Autodesk Fusion 360 part; units mm, degrees
(part 5 of 40)
  line L1833 (198.3385, 89.2864) -> (198.2749, 89.1443) construction
  line L1834 (198.2749, 89.1443) -> (198.2094, 89.0029) construction
  line L1835 (198.2094, 89.0029) -> (198.1418, 88.8621) construction
  line L1836 (198.1418, 88.8621) -> (198.072, 88.7221) construction
  line L1837 (198.072, 88.7221) -> (198.0004, 88.5827) construction
  line L1838 (198.0004, 88.5827) -> (197.927, 88.4439) construction
  line L1839 (197.927, 88.4439) -> (197.8523, 88.3056) construction
  line L1840 (197.8523, 88.3056) -> (197.7763, 88.1678) construction
  line L1841 (197.7763, 88.1678) -> (197.6993, 88.0303) construction
  line L1842 (197.6993, 88.0303) -> (197.6211, 87.8933) construction
  line L1843 (197.6211, 87.8933) -> (197.5416, 87.7568) construction
  line L1844 (197.5416, 87.7568) -> (197.4609, 87.6208) construction
  line L1845 (197.4609, 87.6208) -> (197.379, 87.4852) construction
  line L1846 (197.379, 87.4852) -> (197.2957, 87.3502) construction
  line L1847 (197.2957, 87.3502) -> (197.2112, 87.2157) construction
  line L1848 (197.2112, 87.2157) -> (197.1256, 87.0816) construction
  line L1849 (197.1256, 87.0816) -> (197.0388, 86.948) construction
  line L1850 (197.0388, 86.948) -> (196.951, 86.8148) construction
  line L1851 (196.951, 86.8148) -> (196.8622, 86.682) construction
  line L1852 (196.8622, 86.682) -> (196.7723, 86.5497) construction
  line L1853 (196.7723, 86.5497) -> (196.6814, 86.4179) construction
  line L1854 (196.6814, 86.4179) -> (196.5895, 86.2865) construction
  line L1855 (196.5895, 86.2865) -> (196.4966, 86.1555) construction
  line L1856 (196.4966, 86.1555) -> (196.4027, 86.025) construction
  line L1857 (196.4027, 86.025) -> (196.3078, 85.895) construction
  line L1858 (196.3078, 85.895) -> (196.212, 85.7654) construction
  line L1859 (196.212, 85.7654) -> (196.1152, 85.6362) construction
  line L1860 (196.1152, 85.6362) -> (196.0174, 85.5074) construction
  line L1861 (196.0174, 85.5074) -> (195.9188, 85.3791) construction
  line L1862 (195.9188, 85.3791) -> (195.8193, 85.2512) construction
  line L1863 (195.8193, 85.2512) -> (195.7189, 85.1238) construction
  line L1864 (195.7189, 85.1238) -> (195.6176, 84.9968) construction
  line L1865 (195.6176, 84.9968) -> (195.5154, 84.8702) construction
  line L1866 (195.5154, 84.8702) -> (195.4124, 84.744) construction
  line L1867 (195.4124, 84.744) -> (195.3085, 84.6183) construction
  line L1868 (195.3085, 84.6183) -> (195.2037, 84.493) construction
  line L1869 (195.2037, 84.493) -> (195.0982, 84.3682) construction
  line L1870 (195.0982, 84.3682) -> (194.9918, 84.2438) construction
  line L1871 (194.9918, 84.2438) -> (194.8846, 84.1198) construction
  line L1872 (194.8846, 84.1198) -> (194.7765, 83.9962) construction
  line L1873 (194.7765, 83.9962) -> (194.6677, 83.8731) construction
  line L1874 (194.6677, 83.8731) -> (194.5581, 83.7503) construction
  line L1875 (194.5581, 83.7503) -> (194.4478, 83.6281) construction
  line L1876 (194.4478, 83.6281) -> (194.3366, 83.5062) construction
  line L1877 (194.3366, 83.5062) -> (194.2247, 83.3848) construction
  line L1878 (194.2247, 83.3848) -> (194.112, 83.2638) construction
  line L1879 (194.112, 83.2638) -> (193.9985, 83.1432) construction
  line L1880 (193.9985, 83.1432) -> (193.8843, 83.0231) construction
  line L1881 (193.8843, 83.0231) -> (193.7694, 82.9034) construction
  line L1882 (193.7694, 82.9034) -> (193.6538, 82.7841) construction
  line L1883 (193.6538, 82.7841) -> (193.5374, 82.6653) construction
  line L1884 (193.5374, 82.6653) -> (193.4202, 82.5469) construction
  line L1885 (193.4202, 82.5469) -> (193.3024, 82.4289) construction
  line L1886 (193.3024, 82.4289) -> (193.1839, 82.3113) construction
  line L1887 (193.1839, 82.3113) -> (193.0646, 82.1942) construction
  line L1888 (193.0646, 82.1942) -> (192.9447, 82.0775) construction
  line L1889 (192.9447, 82.0775) -> (192.8241, 81.9612) construction
  line L1890 (192.8241, 81.9612) -> (192.7027, 81.8454) construction
  line L1891 (192.7027, 81.8454) -> (192.5808, 81.73) construction
  line L1892 (192.5808, 81.73) -> (192.4581, 81.615) construction
  line L1893 (192.4581, 81.615) -> (192.3594, 81.5233) construction
  line L1894 (192.3594, 81.5233) -> (192.2851, 81.4548) construction
  line L1895 (192.2851, 81.4548) -> (192.2354, 81.4092) construction
  line L1896 (192.2354, 81.4092) -> (192.2105, 81.3864) construction
  spline S25 degree 5 poles (198.7698, 90.4458) (198.763, 90.4157) (198.7487, 90.3556) (198.7249, 90.2662) (198.6885, 90.1483) (198.6369, 90.0027) (198.5809, 89.8584) (198.5221, 89.7148) (198.4619, 89.5717) (198.4007, 89.4289) (198.3385, 89.2864) (198.2749, 89.1443) (198.2094, 89.0029) (198.1418, 88.8621) (198.072, 88.7221) (198.0004, 88.5827) (197.927, 88.4439) (197.8523, 88.3056) (197.7763, 88.1678) (197.6993, 88.0303) (197.6211, 87.8933) (197.5416, 87.7568) (197.4609, 87.6208) (197.379, 87.4852) (197.2957, 87.3502) (197.2112, 87.2157) (197.1256, 87.0816) (197.0388, 86.948) (196.951, 86.8148) (196.8622, 86.682) (196.7723, 86.5497) (196.6814, 86.4179) (196.5895, 86.2865) (196.4966, 86.1555) (196.4027, 86.025) (196.3078, 85.895) (196.212, 85.7654) (196.1152, 85.6362) (196.0174, 85.5074) (195.9188, 85.3791) (195.8193, 85.2512) (195.7189, 85.1238) (195.6176, 84.9968) (195.5154, 84.8702) (195.4124, 84.744) (195.3085, 84.6183) (195.2037, 84.493) (195.0982, 84.3682) (194.9918, 84.2438) (194.8846, 84.1198) (194.7765, 83.9962) (194.6677, 83.8731) (194.5581, 83.7503) (194.4478, 83.6281) (194.3366, 83.5062) (194.2247, 83.3848) (194.112, 83.2638) (193.9985, 83.1432) (193.8843, 83.0231) (193.7694, 82.9034) (193.6538, 82.7841) (193.5374, 82.6653) (193.4202, 82.5469) (193.3024, 82.4289) (193.1839, 82.3113) (193.0646, 82.1942) (192.9447, 82.0775) (192.8241, 81.9612) (192.7027, 81.8454) (192.5808, 81.73) (192.4581, 81.615) (192.3594, 81.5233) (192.2851, 81.4548) (192.2354, 81.4092) (192.2105, 81.3864) knots 0 0 0 0 0 0 0.01428571 0.02857143 0.04285714 0.05714286 0.07142857 0.08571429 0.1 0.11428571 0.12857143 0.14285714 0.15714286 0.17142857 0.18571429 0.2 0.21428571 0.22857143 0.24285714 0.25714286 0.27142857 0.28571429 0.3 0.31428571 0.32857143 0.34285714 0.35714286 0.37142857 0.38571429 0.4 0.41428571 0.42857143 0.44285714 0.45714286 0.47142857 0.48571429 0.5 0.51428571 0.52857143 0.54285714 0.55714286 0.57142857 0.58571429 0.6 0.61428571 0.62857143 0.64285714 0.65714286 0.67142857 0.68571429 0.7 0.71428571 0.72857143 0.74285714 0.75714286 0.77142857 0.78571429 0.8 0.81428571 0.82857143 0.84285714 0.85714286 0.87142857 0.88571429 0.9 0.91428571 0.92857143 0.94285714 0.95714286 0.97142857 0.98571429 1 1 1 1 1 1
  line L1897 (198.7698, 90.4458) -> (198.763, 90.4157) construction
  line L1898 (198.763, 90.4157) -> (198.7487, 90.3556) construction
  line L1899 (198.7487, 90.3556) -> (198.7249, 90.2662) construction
  line L1900 (198.7249, 90.2662) -> (198.6885, 90.1483) construction
  line L1901 (198.6885, 90.1483) -> (198.6369, 90.0027) construction
  line L1902 (198.6369, 90.0027) -> (198.5809, 89.8584) construction
  line L1903 (198.5809, 89.8584) -> (198.5221, 89.7148) construction
  line L1904 (198.5221, 89.7148) -> (198.4619, 89.5717) construction
  line L1905 (198.4619, 89.5717) -> (198.4007, 89.4289) construction
  line L1906 (198.4007, 89.4289) -> (198.3385, 89.2864) construction
  line L1907 (198.3385, 89.2864) -> (198.2749, 89.1443) construction
  line L1908 (198.2749, 89.1443) -> (198.2094, 89.0029) construction
  line L1909 (198.2094, 89.0029) -> (198.1418, 88.8621) construction
  line L1910 (198.1418, 88.8621) -> (198.072, 88.7221) construction
  line L1911 (198.072, 88.7221) -> (198.0004, 88.5827) construction
  line L1912 (198.0004, 88.5827) -> (197.927, 88.4439) construction
  line L1913 (197.927, 88.4439) -> (197.8523, 88.3056) construction
  line L1914 (197.8523, 88.3056) -> (197.7763, 88.1678) construction
  line L1915 (197.7763, 88.1678) -> (197.6993, 88.0303) construction
  line L1916 (197.6993, 88.0303) -> (197.6211, 87.8933) construction
  line L1917 (197.6211, 87.8933) -> (197.5416, 87.7568) construction
  line L1918 (197.5416, 87.7568) -> (197.4609, 87.6208) construction
  line L1919 (197.4609, 87.6208) -> (197.379, 87.4852) construction
  line L1920 (197.379, 87.4852) -> (197.2957, 87.3502) construction
  line L1921 (197.2957, 87.3502) -> (197.2112, 87.2157) construction
  line L1922 (197.2112, 87.2157) -> (197.1256, 87.0816) construction
  line L1923 (197.1256, 87.0816) -> (197.0388, 86.948) construction
  line L1924 (197.0388, 86.948) -> (196.951, 86.8148) construction
  line L1925 (196.951, 86.8148) -> (196.8622, 86.682) construction
  line L1926 (196.8622, 86.682) -> (196.7723, 86.5497) construction
  line L1927 (196.7723, 86.5497) -> (196.6814, 86.4179) construction
  line L1928 (196.6814, 86.4179) -> (196.5895, 86.2865) construction
  line L1929 (196.5895, 86.2865) -> (196.4966, 86.1555) construction
  line L1930 (196.4966, 86.1555) -> (196.4027, 86.025) construction
  line L1931 (196.4027, 86.025) -> (196.3078, 85.895) construction
  line L1932 (196.3078, 85.895) -> (196.212, 85.7654) construction
  line L1933 (196.212, 85.7654) -> (196.1152, 85.6362) construction
  line L1934 (196.1152, 85.6362) -> (196.0174, 85.5074) construction
  line L1935 (196.0174, 85.5074) -> (195.9188, 85.3791) construction
  line L1936 (195.9188, 85.3791) -> (195.8193, 85.2512) construction
  line L1937 (195.8193, 85.2512) -> (195.7189, 85.1238) construction
  line L1938 (195.7189, 85.1238) -> (195.6176, 84.9968) construction
  line L1939 (195.6176, 84.9968) -> (195.5154, 84.8702) construction
  line L1940 (195.5154, 84.8702) -> (195.4124, 84.744) construction
  line L1941 (195.4124, 84.744) -> (195.3085, 84.6183) construction
  line L1942 (195.3085, 84.6183) -> (195.2037, 84.493) construction
  line L1943 (195.2037, 84.493) -> (195.0982, 84.3682) construction
  line L1944 (195.0982, 84.3682) -> (194.9918, 84.2438) construction
  line L1945 (194.9918, 84.2438) -> (194.8846, 84.1198) construction
  line L1946 (194.8846, 84.1198) -> (194.7765, 83.9962) construction
  line L1947 (194.7765, 83.9962) -> (194.6677, 83.8731) construction
  line L1948 (194.6677, 83.8731) -> (194.5581, 83.7503) construction
  line L1949 (194.5581, 83.7503) -> (194.4478, 83.6281) construction
  line L1950 (194.4478, 83.6281) -> (194.3366, 83.5062) construction
  line L1951 (194.3366, 83.5062) -> (194.2247, 83.3848) construction
  line L1952 (194.2247, 83.3848) -> (194.112, 83.2638) construction
  line L1953 (194.112, 83.2638) -> (193.9985, 83.1432) construction
  line L1954 (193.9985, 83.1432) -> (193.8843, 83.0231) construction
  line L1955 (193.8843, 83.0231) -> (193.7694, 82.9034) construction
  line L1956 (193.7694, 82.9034) -> (193.6538, 82.7841) construction
  line L1957 (193.6538, 82.7841) -> (193.5374, 82.6653) construction
  line L1958 (193.5374, 82.6653) -> (193.4202, 82.5469) construction
  line L1959 (193.4202, 82.5469) -> (193.3024, 82.4289) construction
  line L1960 (193.3024, 82.4289) -> (193.1839, 82.3113) construction
  line L1961 (193.1839, 82.3113) -> (193.0646, 82.1942) construction
  line L1962 (193.0646, 82.1942) -> (192.9447, 82.0775) construction
  line L1963 (192.9447, 82.0775) -> (192.8241, 81.9612) construction
  line L1964 (192.8241, 81.9612) -> (192.7027, 81.8454) construction
  line L1965 (192.7027, 81.8454) -> (192.5808, 81.73) construction
  line L1966 (192.5808, 81.73) -> (192.4581, 81.615) construction
  line L1967 (192.4581, 81.615) -> (192.3594, 81.5233) construction
  line L1968 (192.3594, 81.5233) -> (192.2851, 81.4548) construction
  line L1969 (192.2851, 81.4548) -> (192.2354, 81.4092) construction
  line L1970 (192.2354, 81.4092) -> (192.2105, 81.3864) construction
  arc A68 (170.3188, 110.6216) -> (167.5414, 110.7517) centre (168.8628, 109.2504) ccw
  arc A69 (184.5338, 99.6279) -> (187.6019, 98.0646) centre (212.132, 150) ccw
  line L1971 (188.5839, 95.4634) -> (187.9372, 93.9655)
  arc A70 (199.127, 207.9623) -> (201.4504, 206.435) centre (201.0785, 208.4001) ccw
  line L1972 (188.5839, 95.4634) -> (187.9372, 93.9655)
  arc A71 (184.5338, 99.6279) -> (187.6019, 98.0646) centre (212.132, 150) ccw
  spline S26 degree 5 poles (198.7698, 209.5542) (198.763, 209.5843) (198.7487, 209.6444) (198.7249, 209.7338) (198.6885, 209.8517) (198.6369, 209.9973) (198.5809, 210.1416) (198.5221, 210.2852) (198.4619, 210.4283) (198.4007, 210.5711) (198.3385, 210.7136) (198.2749, 210.8557) (198.2094, 210.9971) (198.1418, 211.1379) (198.072, 211.2779) (198.0004, 211.4173) (197.927, 211.5561) (197.8523, 211.6944) (197.7763, 211.8322) (197.6993, 211.9697) (197.6211, 212.1067) (197.5416, 212.2432) (197.4609, 212.3792) (197.379, 212.5148) (197.2957, 212.6498) (197.2112, 212.7843) (197.1256, 212.9184) (197.0388, 213.052) (196.951, 213.1852) (196.8622, 213.318) (196.7723, 213.4503) (196.6814, 213.5821) (196.5895, 213.7135) (196.4966, 213.8445) (196.4027, 213.975) (196.3078, 214.105) (196.212, 214.2346) (196.1152, 214.3638) (196.0174, 214.4926) (195.9188, 214.6209) (195.8193, 214.7488) (195.7189, 214.8762) (195.6176, 215.0032) (195.5154, 215.1298) (195.4124, 215.256) (195.3085, 215.3817) (195.2037, 215.507) (195.0982, 215.6318) (194.9918, 215.7562) (194.8846, 215.8802) (194.7765, 216.0038) (194.6677, 216.1269) (194.5581, 216.2497) (194.4478, 216.3719) (194.3366, 216.4938) (194.2247, 216.6152) (194.112, 216.7362) (193.9985, 216.8568) (193.8843, 216.9769) (193.7694, 217.0966) (193.6538, 217.2159) (193.5374, 217.3347) (193.4202, 217.4531) (193.3024, 217.5711) (193.1839, 217.6887) (193.0646, 217.8058) (192.9447, 217.9225) (192.8241, 218.0388) (192.7027, 218.1546) (192.5808, 218.27) (192.4581, 218.385) (192.3594, 218.4767) (192.2851, 218.5452) (192.2354, 218.5908) (192.2105, 218.6136) knots 0 0 0 0 0 0 0.01428571 0.02857143 0.04285714 0.05714286 0.07142857 0.08571429 0.1 0.11428571 0.12857143 0.14285714 0.15714286 0.17142857 0.18571429 0.2 0.21428571 0.22857143 0.24285714 0.25714286 0.27142857 0.28571429 0.3 0.31428571 0.32857143 0.34285714 0.35714286 0.37142857 0.38571429 0.4 0.41428571 0.42857143 0.44285714 0.45714286 0.47142857 0.48571429 0.5 0.51428571 0.52857143 0.54285714 0.55714286 0.57142857 0.58571429 0.6 0.61428571 0.62857143 0.64285714 0.65714286 0.67142857 0.68571429 0.7 0.71428571 0.72857143 0.74285714 0.75714286 0.77142857 0.78571429 0.8 0.81428571 0.82857143 0.84285714 0.85714286 0.87142857 0.88571429 0.9 0.91428571 0.92857143 0.94285714 0.95714286 0.97142857 0.98571429 1 1 1 1 1 1
  line L1973 (198.7698, 209.5542) -> (198.763, 209.5843) construction
  line L1974 (198.763, 209.5843) -> (198.7487, 209.6444) construction
  line L1975 (198.7487, 209.6444) -> (198.7249, 209.7338) construction
  line L1976 (198.7249, 209.7338) -> (198.6885, 209.8517) construction
  line L1977 (198.6885, 209.8517) -> (198.6369, 209.9973) construction
  line L1978 (198.6369, 209.9973) -> (198.5809, 210.1416) construction
  line L1979 (198.5809, 210.1416) -> (198.5221, 210.2852) construction
  line L1980 (198.5221, 210.2852) -> (198.4619, 210.4283) construction
  line L1981 (198.4619, 210.4283) -> (198.4007, 210.5711) construction
  line L1982 (198.4007, 210.5711) -> (198.3385, 210.7136) construction
  line L1983 (198.3385, 210.7136) -> (198.2749, 210.8557) construction
  line L1984 (198.2749, 210.8557) -> (198.2094, 210.9971) construction
  line L1985 (198.2094, 210.9971) -> (198.1418, 211.1379) construction
  line L1986 (198.1418, 211.1379) -> (198.072, 211.2779) construction
  line L1987 (198.072, 211.2779) -> (198.0004, 211.4173) construction
  line L1988 (198.0004, 211.4173) -> (197.927, 211.5561) construction
  line L1989 (197.927, 211.5561) -> (197.8523, 211.6944) construction
  line L1990 (197.8523, 211.6944) -> (197.7763, 211.8322) construction
  line L1991 (197.7763, 211.8322) -> (197.6993, 211.9697) construction
  line L1992 (197.6993, 211.9697) -> (197.6211, 212.1067) construction
  line L1993 (197.6211, 212.1067) -> (197.5416, 212.2432) construction
  line L1994 (197.5416, 212.2432) -> (197.4609, 212.3792) construction
  line L1995 (197.4609, 212.3792) -> (197.379, 212.5148) construction
  line L1996 (197.379, 212.5148) -> (197.2957, 212.6498) construction
  line L1997 (197.2957, 212.6498) -> (197.2112, 212.7843) construction
  line L1998 (197.2112, 212.7843) -> (197.1256, 212.9184) construction
  line L1999 (197.1256, 212.9184) -> (197.0388, 213.052) construction
  line L2000 (197.0388, 213.052) -> (196.951, 213.1852) construction
  line L2001 (196.951, 213.1852) -> (196.8622, 213.318) construction
  line L2002 (196.8622, 213.318) -> (196.7723, 213.4503) construction
  line L2003 (196.7723, 213.4503) -> (196.6814, 213.5821) construction
  line L2004 (196.6814, 213.5821) -> (196.5895, 213.7135) construction
  line L2005 (196.5895, 213.7135) -> (196.4966, 213.8445) construction
  line L2006 (196.4966, 213.8445) -> (196.4027, 213.975) construction
  line L2007 (196.4027, 213.975) -> (196.3078, 214.105) construction
  line L2008 (196.3078, 214.105) -> (196.212, 214.2346) construction
  line L2009 (196.212, 214.2346) -> (196.1152, 214.3638) construction
  line L2010 (196.1152, 214.3638) -> (196.0174, 214.4926) construction
  line L2011 (196.0174, 214.4926) -> (195.9188, 214.6209) construction
  line L2012 (195.9188, 214.6209) -> (195.8193, 214.7488) construction
  line L2013 (195.8193, 214.7488) -> (195.7189, 214.8762) construction
  line L2014 (195.7189, 214.8762) -> (195.6176, 215.0032) construction
  line L2015 (195.6176, 215.0032) -> (195.5154, 215.1298) construction
  line L2016 (195.5154, 215.1298) -> (195.4124, 215.256) construction
  line L2017 (195.4124, 215.256) -> (195.3085, 215.3817) construction
  line L2018 (195.3085, 215.3817) -> (195.2037, 215.507) construction
  line L2019 (195.2037, 215.507) -> (195.0982, 215.6318) construction
  line L2020 (195.0982, 215.6318) -> (194.9918, 215.7562) construction
  line L2021 (194.9918, 215.7562) -> (194.8846, 215.8802) construction
  line L2022 (194.8846, 215.8802) -> (194.7765, 216.0038) construction
  line L2023 (194.7765, 216.0038) -> (194.6677, 216.1269) construction
  line L2024 (194.6677, 216.1269) -> (194.5581, 216.2497) construction
  line L2025 (194.5581, 216.2497) -> (194.4478, 216.3719) construction
  line L2026 (194.4478, 216.3719) -> (194.3366, 216.4938) construction
  line L2027 (194.3366, 216.4938) -> (194.2247, 216.6152) construction
  line L2028 (194.2247, 216.6152) -> (194.112, 216.7362) construction
  line L2029 (194.112, 216.7362) -> (193.9985, 216.8568) construction
  line L2030 (193.9985, 216.8568) -> (193.8843, 216.9769) construction
  line L2031 (193.8843, 216.9769) -> (193.7694, 217.0966) construction
  line L2032 (193.7694, 217.0966) -> (193.6538, 217.2159) construction
  line L2033 (193.6538, 217.2159) -> (193.5374, 217.3347) construction
  line L2034 (193.5374, 217.3347) -> (193.4202, 217.4531) construction
  line L2035 (193.4202, 217.4531) -> (193.3024, 217.5711) construction
  line L2036 (193.3024, 217.5711) -> (193.1839, 217.6887) construction
  line L2037 (193.1839, 217.6887) -> (193.0646, 217.8058) construction
  line L2038 (193.0646, 217.8058) -> (192.9447, 217.9225) construction
  line L2039 (192.9447, 217.9225) -> (192.8241, 218.0388) construction
  line L2040 (192.8241, 218.0388) -> (192.7027, 218.1546) construction
  line L2041 (192.7027, 218.1546) -> (192.5808, 218.27) construction
  line L2042 (192.5808, 218.27) -> (192.4581, 218.385) construction
  line L2043 (192.4581, 218.385) -> (192.3594, 218.4767) construction
  line L2044 (192.3594, 218.4767) -> (192.2851, 218.5452) construction
  line L2045 (192.2851, 218.5452) -> (192.2354, 218.5908) construction
  line L2046 (192.2354, 218.5908) -> (192.2105, 218.6136) construction
  arc A72 (188.5839, 95.4634) -> (187.6019, 98.0646) centre (186.7478, 96.2562) ccw
  spline S27 degree 5 poles (198.7698, 209.5542) (198.763, 209.5843) (198.7487, 209.6444) (198.7249, 209.7338) (198.6885, 209.8517) (198.6369, 209.9973) (198.5809, 210.1416) (198.5221, 210.2852) (198.4619, 210.4283) (198.4007, 210.5711) (198.3385, 210.7136) (198.2749, 210.8557) (198.2094, 210.9971) (198.1418, 211.1379) (198.072, 211.2779) (198.0004, 211.4173) (197.927, 211.5561) (197.8523, 211.6944) (197.7763, 211.8322) (197.6993, 211.9697) (197.6211, 212.1067) (197.5416, 212.2432) (197.4609, 212.3792) (197.379, 212.5148) (197.2957, 212.6498) (197.2112, 212.7843) (197.1256, 212.9184) (197.0388, 213.052) (196.951, 213.1852) (196.8622, 213.318) (196.7723, 213.4503) (196.6814, 213.5821) (196.5895, 213.7135) (196.4966, 213.8445) (196.4027, 213.975) (196.3078, 214.105) (196.212, 214.2346) (196.1152, 214.3638) (196.0174, 214.4926) (195.9188, 214.6209) (195.8193, 214.7488) (195.7189, 214.8762) (195.6176, 215.0032) (195.5154, 215.1298) (195.4124, 215.256) (195.3085, 215.3817) (195.2037, 215.507) (195.0982, 215.6318) (194.9918, 215.7562) (194.8846, 215.8802) (194.7765, 216.0038) (194.6677, 216.1269) (194.5581, 216.2497) (194.4478, 216.3719) (194.3366, 216.4938) (194.2247, 216.6152) (194.112, 216.7362) (193.9985, 216.8568) (193.8843, 216.9769) (193.7694, 217.0966) (193.6538, 217.2159) (193.5374, 217.3347) (193.4202, 217.4531) (193.3024, 217.5711) (193.1839, 217.6887) (193.0646, 217.8058) (192.9447, 217.9225) (192.8241, 218.0388) (192.7027, 218.1546) (192.5808, 218.27) (192.4581, 218.385) (192.3594, 218.4767) (192.2851, 218.5452) (192.2354, 218.5908) (192.2105, 218.6136) knots 0 0 0 0 0 0 0.01428571 0.02857143 0.04285714 0.05714286 0.07142857 0.08571429 0.1 0.11428571 0.12857143 0.14285714 0.15714286 0.17142857 0.18571429 0.2 0.21428571 0.22857143 0.24285714 0.25714286 0.27142857 0.28571429 0.3 0.31428571 0.32857143 0.34285714 0.35714286 0.37142857 0.38571429 0.4 0.41428571 0.42857143 0.44285714 0.45714286 0.47142857 0.48571429 0.5 0.51428571 0.52857143 0.54285714 0.55714286 0.57142857 0.58571429 0.6 0.61428571 0.62857143 0.64285714 0.65714286 0.67142857 0.68571429 0.7 0.71428571 0.72857143 0.74285714 0.75714286 0.77142857 0.78571429 0.8 0.81428571 0.82857143 0.84285714 0.85714286 0.87142857 0.88571429 0.9 0.91428571 0.92857143 0.94285714 0.95714286 0.97142857 0.98571429 1 1 1 1 1 1
  line L2047 (198.7698, 209.5542) -> (198.763, 209.5843) construction
  line L2048 (198.763, 209.5843) -> (198.7487, 209.6444) construction
  line L2049 (198.7487, 209.6444) -> (198.7249, 209.7338) construction
  line L2050 (198.7249, 209.7338) -> (198.6885, 209.8517) construction
  line L2051 (198.6885, 209.8517) -> (198.6369, 209.9973) construction
  line L2052 (198.6369, 209.9973) -> (198.5809, 210.1416) construction
  line L2053 (198.5809, 210.1416) -> (198.5221, 210.2852) construction
  line L2054 (198.5221, 210.2852) -> (198.4619, 210.4283) construction
  line L2055 (198.4619, 210.4283) -> (198.4007, 210.5711) construction
  line L2056 (198.4007, 210.5711) -> (198.3385, 210.7136) construction
  line L2057 (198.3385, 210.7136) -> (198.2749, 210.8557) construction
  line L2058 (198.2749, 210.8557) -> (198.2094, 210.9971) construction
  line L2059 (198.2094, 210.9971) -> (198.1418, 211.1379) construction
  line L2060 (198.1418, 211.1379) -> (198.072, 211.2779) construction
  line L2061 (198.072, 211.2779) -> (198.0004, 211.4173) construction
  line L2062 (198.0004, 211.4173) -> (197.927, 211.5561) construction
  line L2063 (197.927, 211.5561) -> (197.8523, 211.6944) construction
  line L2064 (197.8523, 211.6944) -> (197.7763, 211.8322) construction
  line L2065 (197.7763, 211.8322) -> (197.6993, 211.9697) construction
  line L2066 (197.6993, 211.9697) -> (197.6211, 212.1067) construction
  line L2067 (197.6211, 212.1067) -> (197.5416, 212.2432) construction
  line L2068 (197.5416, 212.2432) -> (197.4609, 212.3792) construction
  line L2069 (197.4609, 212.3792) -> (197.379, 212.5148) construction
  line L2070 (197.379, 212.5148) -> (197.2957, 212.6498) construction
  line L2071 (197.2957, 212.6498) -> (197.2112, 212.7843) construction
  line L2072 (197.2112, 212.7843) -> (197.1256, 212.9184) construction
  line L2073 (197.1256, 212.9184) -> (197.0388, 213.052) construction
  line L2074 (197.0388, 213.052) -> (196.951, 213.1852) construction
  line L2075 (196.951, 213.1852) -> (196.8622, 213.318) construction
  line L2076 (196.8622, 213.318) -> (196.7723, 213.4503) construction
  line L2077 (196.7723, 213.4503) -> (196.6814, 213.5821) construction
  line L2078 (196.6814, 213.5821) -> (196.5895, 213.7135) construction
  line L2079 (196.5895, 213.7135) -> (196.4966, 213.8445) construction
  line L2080 (196.4966, 213.8445) -> (196.4027, 213.975) construction
  line L2081 (196.4027, 213.975) -> (196.3078, 214.105) construction
  line L2082 (196.3078, 214.105) -> (196.212, 214.2346) construction
  line L2083 (196.212, 214.2346) -> (196.1152, 214.3638) construction
  line L2084 (196.1152, 214.3638) -> (196.0174, 214.4926) construction
  line L2085 (196.0174, 214.4926) -> (195.9188, 214.6209) construction
  line L2086 (195.9188, 214.6209) -> (195.8193, 214.7488) construction
  line L2087 (195.8193, 214.7488) -> (195.7189, 214.8762) construction
  line L2088 (195.7189, 214.8762) -> (195.6176, 215.0032) construction
  line L2089 (195.6176, 215.0032) -> (195.5154, 215.1298) construction
  line L2090 (195.5154, 215.1298) -> (195.4124, 215.256) construction
  line L2091 (195.4124, 215.256) -> (195.3085, 215.3817) construction
  line L2092 (195.3085, 215.3817) -> (195.2037, 215.507) construction
  line L2093 (195.2037, 215.507) -> (195.0982, 215.6318) construction
  line L2094 (195.0982, 215.6318) -> (194.9918, 215.7562) construction
  line L2095 (194.9918, 215.7562) -> (194.8846, 215.8802) construction
  line L2096 (194.8846, 215.8802) -> (194.7765, 216.0038) construction
  line L2097 (194.7765, 216.0038) -> (194.6677, 216.1269) construction
  line L2098 (194.6677, 216.1269) -> (194.5581, 216.2497) construction
  line L2099 (194.5581, 216.2497) -> (194.4478, 216.3719) construction
  line L2100 (194.4478, 216.3719) -> (194.3366, 216.4938) construction
  line L2101 (194.3366, 216.4938) -> (194.2247, 216.6152) construction
  line L2102 (194.2247, 216.6152) -> (194.112, 216.7362) construction
  line L2103 (194.112, 216.7362) -> (193.9985, 216.8568) construction
  line L2104 (193.9985, 216.8568) -> (193.8843, 216.9769) construction
  line L2105 (193.8843, 216.9769) -> (193.7694, 217.0966) construction
  line L2106 (193.7694, 217.0966) -> (193.6538, 217.2159) construction
  line L2107 (193.6538, 217.2159) -> (193.5374, 217.3347) construction
  line L2108 (193.5374, 217.3347) -> (193.4202, 217.4531) construction
  line L2109 (193.4202, 217.4531) -> (193.3024, 217.5711) construction
  line L2110 (193.3024, 217.5711) -> (193.1839, 217.6887) construction
  line L2111 (193.1839, 217.6887) -> (193.0646, 217.8058) construction
  line L2112 (193.0646, 217.8058) -> (192.9447, 217.9225) construction
  line L2113 (192.9447, 217.9225) -> (192.8241, 218.0388) construction
  line L2114 (192.8241, 218.0388) -> (192.7027, 218.1546) construction
  line L2115 (192.7027, 218.1546) -> (192.5808, 218.27) construction
  line L2116 (192.5808, 218.27) -> (192.4581, 218.385) construction
  line L2117 (192.4581, 218.385) -> (192.3594, 218.4767) construction
  line L2118 (192.3594, 218.4767) -> (192.2851, 218.5452) construction
  line L2119 (192.2851, 218.5452) -> (192.2354, 218.5908) construction
  line L2120 (192.2354, 218.5908) -> (192.2105, 218.6136) construction
  line L2121 (270.0943, 136.995) -> (271.6862, 136.6378)
  arc A73 (188.5839, 95.4634) -> (187.6019, 98.0646) centre (186.7478, 96.2562) ccw
  arc A74 (268.567, 139.3184) -> (270.0943, 136.995) centre (270.5321, 138.9465) ccw
  arc A75 (170.3188, 110.6216) -> (167.5414, 110.7517) centre (168.8628, 109.2504) ccw
  arc A76 (268.567, 139.3184) -> (270.0943, 136.995) centre (270.5321, 138.9465) ccw
  arc A77 (170.3188, 110.6216) -> (172.7536, 108.1868) centre (212.132, 150) ccw
  line L2122 (270.0943, 136.995) -> (271.6862, 136.6378)
  arc A78 (170.3188, 110.6216) -> (172.7536, 108.1868) centre (212.132, 150) ccw
  spline S28 degree 5 poles (217.8271, 89.2315) (217.8299, 89.2007) (217.8349, 89.1391) (217.8398, 89.0467) (217.8417, 88.9234) (217.8376, 88.769) (217.8289, 88.6144) (217.8174, 88.4597) (217.8043, 88.305) (217.7903, 88.1502) (217.7751, 87.9955) (217.7585, 87.8407) (217.74, 87.686) (217.7191, 87.5312) (217.6961, 87.3765) (217.671, 87.2218) (217.6441, 87.0671) (217.6158, 86.9125) (217.5862, 86.7579) (217.5553, 86.6034) (217.5233, 86.4489) (217.4899, 86.2945) (217.4552, 86.1402) (217.4191, 85.986) (217.3817, 85.8318) (217.3429, 85.6778) (217.3029, 85.5238) (217.2617, 85.3699) (217.2193, 85.2161) (217.1759, 85.0624) (217.1313, 84.9088) (217.0856, 84.7553) (217.0388, 84.602) (216.9909, 84.4487) (216.9419, 84.2956) (216.8919, 84.1426) (216.8407, 83.9897) (216.7886, 83.8369) (216.7355, 83.6842) (216.6813, 83.5317) (216.6262, 83.3794) (216.57, 83.2271) (216.513, 83.075) (216.4549, 82.923) (216.3959, 82.7712) (216.3359, 82.6196) (216.275, 82.468) (216.2132, 82.3167) (216.1505, 82.1655) (216.0868, 82.0144) (216.0223, 81.8635) (215.9569, 81.7128) (215.8905, 81.5622) (215.8233, 81.4118) (215.7553, 81.2616) (215.6863, 81.1115) (215.6166, 80.9616) (215.5459, 80.8119) (215.4745, 80.6624) (215.4021, 80.513) (215.329, 80.3638) (215.255, 80.2148) (215.1802, 80.066) (215.1046, 79.9174) (215.0282, 79.7689) (214.951, 79.6207) (214.873, 79.4726) (214.7942, 79.3248) (214.7146, 79.1771) (214.6343, 79.0297) (214.5531, 78.8824) (214.4876, 78.7648) (214.4381, 78.6766) (214.4049, 78.6179) (214.3883, 78.5885) knots 0 0 0 0 0 0 0.01428571 0.02857143 0.04285714 0.05714286 0.07142857 0.08571429 0.1 0.11428571 0.12857143 0.14285714 0.15714286 0.17142857 0.18571429 0.2 0.21428571 0.22857143 0.24285714 0.25714286 0.27142857 0.28571429 0.3 0.31428571 0.32857143 0.34285714 0.35714286 0.37142857 0.38571429 0.4 0.41428571 0.42857143 0.44285714 0.45714286 0.47142857 0.48571429 0.5 0.51428571 0.52857143 0.54285714 0.55714286 0.57142857 0.58571429 0.6 0.61428571 0.62857143 0.64285714 0.65714286 0.67142857 0.68571429 0.7 0.71428571 0.72857143 0.74285714 0.75714286 0.77142857 0.78571429 0.8 0.81428571 0.82857143 0.84285714 0.85714286 0.87142857 0.88571429 0.9 0.91428571 0.92857143 0.94285714 0.95714286 0.97142857 0.98571429 1 1 1 1 1 1
  line L2123 (217.8271, 89.2315) -> (217.8299, 89.2007) construction
  line L2124 (217.8299, 89.2007) -> (217.8349, 89.1391) construction
  line L2125 (217.8349, 89.1391) -> (217.8398, 89.0467) construction
  line L2126 (217.8398, 89.0467) -> (217.8417, 88.9234) construction
  line L2127 (217.8417, 88.9234) -> (217.8376, 88.769) construction
  line L2128 (217.8376, 88.769) -> (217.8289, 88.6144) construction
  line L2129 (217.8289, 88.6144) -> (217.8174, 88.4597) construction
  line L2130 (217.8174, 88.4597) -> (217.8043, 88.305) construction
  line L2131 (217.8043, 88.305) -> (217.7903, 88.1502) construction
  line L2132 (217.7903, 88.1502) -> (217.7751, 87.9955) construction
  line L2133 (217.7751, 87.9955) -> (217.7585, 87.8407) construction
  line L2134 (217.7585, 87.8407) -> (217.74, 87.686) construction
  line L2135 (217.74, 87.686) -> (217.7191, 87.5312) construction
  line L2136 (217.7191, 87.5312) -> (217.6961, 87.3765) construction
  line L2137 (217.6961, 87.3765) -> (217.671, 87.2218) construction
  line L2138 (217.671, 87.2218) -> (217.6441, 87.0671) construction
  line L2139 (217.6441, 87.0671) -> (217.6158, 86.9125) construction
  line L2140 (217.6158, 86.9125) -> (217.5862, 86.7579) construction
  line L2141 (217.5862, 86.7579) -> (217.5553, 86.6034) construction
  line L2142 (217.5553, 86.6034) -> (217.5233, 86.4489) construction
  line L2143 (217.5233, 86.4489) -> (217.4899, 86.2945) construction
  line L2144 (217.4899, 86.2945) -> (217.4552, 86.1402) construction
  line L2145 (217.4552, 86.1402) -> (217.4191, 85.986) construction
  line L2146 (217.4191, 85.986) -> (217.3817, 85.8318) construction
  line L2147 (217.3817, 85.8318) -> (217.3429, 85.6778) construction
  line L2148 (217.3429, 85.6778) -> (217.3029, 85.5238) construction
  line L2149 (217.3029, 85.5238) -> (217.2617, 85.3699) construction
  line L2150 (217.2617, 85.3699) -> (217.2193, 85.2161) construction
  line L2151 (217.2193, 85.2161) -> (217.1759, 85.0624) construction
  line L2152 (217.1759, 85.0624) -> (217.1313, 84.9088) construction
  line L2153 (217.1313, 84.9088) -> (217.0856, 84.7553) construction
  line L2154 (217.0856, 84.7553) -> (217.0388, 84.602) construction
  line L2155 (217.0388, 84.602) -> (216.9909, 84.4487) construction
  line L2156 (216.9909, 84.4487) -> (216.9419, 84.2956) construction
  line L2157 (216.9419, 84.2956) -> (216.8919, 84.1426) construction
  line L2158 (216.8919, 84.1426) -> (216.8407, 83.9897) construction
  line L2159 (216.8407, 83.9897) -> (216.7886, 83.8369) construction
  line L2160 (216.7886, 83.8369) -> (216.7355, 83.6842) construction
  line L2161 (216.7355, 83.6842) -> (216.6813, 83.5317) construction
  line L2162 (216.6813, 83.5317) -> (216.6262, 83.3794) construction
  line L2163 (216.6262, 83.3794) -> (216.57, 83.2271) construction
  line L2164 (216.57, 83.2271) -> (216.513, 83.075) construction
  line L2165 (216.513, 83.075) -> (216.4549, 82.923) construction
  line L2166 (216.4549, 82.923) -> (216.3959, 82.7712) construction
  line L2167 (216.3959, 82.7712) -> (216.3359, 82.6196) construction
  line L2168 (216.3359, 82.6196) -> (216.275, 82.468) construction
  line L2169 (216.275, 82.468) -> (216.2132, 82.3167) construction
  line L2170 (216.2132, 82.3167) -> (216.1505, 82.1655) construction
  line L2171 (216.1505, 82.1655) -> (216.0868, 82.0144) construction
  line L2172 (216.0868, 82.0144) -> (216.0223, 81.8635) construction
  line L2173 (216.0223, 81.8635) -> (215.9569, 81.7128) construction
  line L2174 (215.9569, 81.7128) -> (215.8905, 81.5622) construction
  line L2175 (215.8905, 81.5622) -> (215.8233, 81.4118) construction
  line L2176 (215.8233, 81.4118) -> (215.7553, 81.2616) construction
  line L2177 (215.7553, 81.2616) -> (215.6863, 81.1115) construction
  line L2178 (215.6863, 81.1115) -> (215.6166, 80.9616) construction
  line L2179 (215.6166, 80.9616) -> (215.5459, 80.8119) construction
  line L2180 (215.5459, 80.8119) -> (215.4745, 80.6624) construction
  line L2181 (215.4745, 80.6624) -> (215.4021, 80.513) construction
  line L2182 (215.4021, 80.513) -> (215.329, 80.3638) construction
  line L2183 (215.329, 80.3638) -> (215.255, 80.2148) construction
  line L2184 (215.255, 80.2148) -> (215.1802, 80.066) construction
  line L2185 (215.1802, 80.066) -> (215.1046, 79.9174) construction
  line L2186 (215.1046, 79.9174) -> (215.0282, 79.7689) construction
  line L2187 (215.0282, 79.7689) -> (214.951, 79.6207) construction
  line L2188 (214.951, 79.6207) -> (214.873, 79.4726) construction
  line L2189 (214.873, 79.4726) -> (214.7942, 79.3248) construction
  line L2190 (214.7942, 79.3248) -> (214.7146, 79.1771) construction
  line L2191 (214.7146, 79.1771) -> (214.6343, 79.0297) construction
  line L2192 (214.6343, 79.0297) -> (214.5531, 78.8824) construction
  line L2193 (214.5531, 78.8824) -> (214.4876, 78.7648) construction
  line L2194 (214.4876, 78.7648) -> (214.4381, 78.6766) construction
  line L2195 (214.4381, 78.6766) -> (214.4049, 78.6179) construction
  line L2196 (214.4049, 78.6179) -> (214.3883, 78.5885) construction
  spline S29 degree 5 poles (217.8271, 89.2315) (217.8299, 89.2007) (217.8349, 89.1391) (217.8398, 89.0467) (217.8417, 88.9234) (217.8376, 88.769) (217.8289, 88.6144) (217.8174, 88.4597) (217.8043, 88.305) (217.7903, 88.1502) (217.7751, 87.9955) (217.7585, 87.8407) (217.74, 87.686) (217.7191, 87.5312) (217.6961, 87.3765) (217.671, 87.2218) (217.6441, 87.0671) (217.6158, 86.9125) (217.5862, 86.7579) (217.5553, 86.6034) (217.5233, 86.4489) (217.4899, 86.2945) (217.4552, 86.1402) (217.4191, 85.986) (217.3817, 85.8318) (217.3429, 85.6778) (217.3029, 85.5238) (217.2617, 85.3699) (217.2193, 85.2161) (217.1759, 85.0624) (217.1313, 84.9088) (217.0856, 84.7553) (217.0388, 84.602) (216.9909, 84.4487) (216.9419, 84.2956) (216.8919, 84.1426) (216.8407, 83.9897) (216.7886, 83.8369) (216.7355, 83.6842) (216.6813, 83.5317) (216.6262, 83.3794) (216.57, 83.2271) (216.513, 83.075) (216.4549, 82.923) (216.3959, 82.7712) (216.3359, 82.6196) (216.275, 82.468) (216.2132, 82.3167) (216.1505, 82.1655) (216.0868, 82.0144) (216.0223, 81.8635) (215.9569, 81.7128) (215.8905, 81.5622) (215.8233, 81.4118) (215.7553, 81.2616) (215.6863, 81.1115) (215.6166, 80.9616) (215.5459, 80.8119) (215.4745, 80.6624) (215.4021, 80.513) (215.329, 80.3638) (215.255, 80.2148) (215.1802, 80.066) (215.1046, 79.9174) (215.0282, 79.7689) (214.951, 79.6207) (214.873, 79.4726) (214.7942, 79.3248) (214.7146, 79.1771) (214.6343, 79.0297) (214.5531, 78.8824) (214.4876, 78.7648) (214.4381, 78.6766) (214.4049, 78.6179) (214.3883, 78.5885) knots 0 0 0 0 0 0 0.01428571 0.02857143 0.04285714 0.05714286 0.07142857 0.08571429 0.1 0.11428571 0.12857143 0.14285714 0.15714286 0.17142857 0.18571429 0.2 0.21428571 0.22857143 0.24285714 0.25714286 0.27142857 0.28571429 0.3 0.31428571 0.32857143 0.34285714 0.35714286 0.37142857 0.38571429 0.4 0.41428571 0.42857143 0.44285714 0.45714286 0.47142857 0.48571429 0.5 0.51428571 0.52857143 0.54285714 0.55714286 0.57142857 0.58571429 0.6 0.61428571 0.62857143 0.64285714 0.65714286 0.67142857 0.68571429 0.7 0.71428571 0.72857143 0.74285714 0.75714286 0.77142857 0.78571429 0.8 0.81428571 0.82857143 0.84285714 0.85714286 0.87142857 0.88571429 0.9 0.91428571 0.92857143 0.94285714 0.95714286 0.97142857 0.98571429 1 1 1 1 1 1
  line L2197 (217.8271, 89.2315) -> (217.8299, 89.2007) construction
  line L2198 (217.8299, 89.2007) -> (217.8349, 89.1391) construction
  line L2199 (217.8349, 89.1391) -> (217.8398, 89.0467) construction
  line L2200 (217.8398, 89.0467) -> (217.8417, 88.9234) construction
  line L2201 (217.8417, 88.9234) -> (217.8376, 88.769) construction
  line L2202 (217.8376, 88.769) -> (217.8289, 88.6144) construction
  line L2203 (217.8289, 88.6144) -> (217.8174, 88.4597) construction
  line L2204 (217.8174, 88.4597) -> (217.8043, 88.305) construction
  line L2205 (217.8043, 88.305) -> (217.7903, 88.1502) construction
  line L2206 (217.7903, 88.1502) -> (217.7751, 87.9955) construction
  line L2207 (217.7751, 87.9955) -> (217.7585, 87.8407) construction
  line L2208 (217.7585, 87.8407) -> (217.74, 87.686) construction
  line L2209 (217.74, 87.686) -> (217.7191, 87.5312) construction
  line L2210 (217.7191, 87.5312) -> (217.6961, 87.3765) construction
  line L2211 (217.6961, 87.3765) -> (217.671, 87.2218) construction
  line L2212 (217.671, 87.2218) -> (217.6441, 87.0671) construction
  line L2213 (217.6441, 87.0671) -> (217.6158, 86.9125) construction
  line L2214 (217.6158, 86.9125) -> (217.5862, 86.7579) construction
  line L2215 (217.5862, 86.7579) -> (217.5553, 86.6034) construction
  line L2216 (217.5553, 86.6034) -> (217.5233, 86.4489) construction
  line L2217 (217.5233, 86.4489) -> (217.4899, 86.2945) construction
  line L2218 (217.4899, 86.2945) -> (217.4552, 86.1402) construction
  line L2219 (217.4552, 86.1402) -> (217.4191, 85.986) construction
  line L2220 (217.4191, 85.986) -> (217.3817, 85.8318) construction
  line L2221 (217.3817, 85.8318) -> (217.3429, 85.6778) construction
  line L2222 (217.3429, 85.6778) -> (217.3029, 85.5238) construction
  line L2223 (217.3029, 85.5238) -> (217.2617, 85.3699) construction
  line L2224 (217.2617, 85.3699) -> (217.2193, 85.2161) construction
  line L2225 (217.2193, 85.2161) -> (217.1759, 85.0624) construction
  line L2226 (217.1759, 85.0624) -> (217.1313, 84.9088) construction
  line L2227 (217.1313, 84.9088) -> (217.0856, 84.7553) construction
  line L2228 (217.0856, 84.7553) -> (217.0388, 84.602) construction
  line L2229 (217.0388, 84.602) -> (216.9909, 84.4487) construction
  line L2230 (216.9909, 84.4487) -> (216.9419, 84.2956) construction
  line L2231 (216.9419, 84.2956) -> (216.8919, 84.1426) construction
  line L2232 (216.8919, 84.1426) -> (216.8407, 83.9897) construction
  line L2233 (216.8407, 83.9897) -> (216.7886, 83.8369) construction
  line L2234 (216.7886, 83.8369) -> (216.7355, 83.6842) construction
  line L2235 (216.7355, 83.6842) -> (216.6813, 83.5317) construction
  line L2236 (216.6813, 83.5317) -> (216.6262, 83.3794) construction
  line L2237 (216.6262, 83.3794) -> (216.57, 83.2271) construction
  line L2238 (216.57, 83.2271) -> (216.513, 83.075) construction
  line L2239 (216.513, 83.075) -> (216.4549, 82.923) construction
  line L2240 (216.4549, 82.923) -> (216.3959, 82.7712) construction
  line L2241 (216.3959, 82.7712) -> (216.3359, 82.6196) construction
  line L2242 (216.3359, 82.6196) -> (216.275, 82.468) construction
  line L2243 (216.275, 82.468) -> (216.2132, 82.3167) construction
  line L2244 (216.2132, 82.3167) -> (216.1505, 82.1655) construction
  line L2245 (216.1505, 82.1655) -> (216.0868, 82.0144) construction
  line L2246 (216.0868, 82.0144) -> (216.0223, 81.8635) construction
  line L2247 (216.0223, 81.8635) -> (215.9569, 81.7128) construction
  line L2248 (215.9569, 81.7128) -> (215.8905, 81.5622) construction
  line L2249 (215.8905, 81.5622) -> (215.8233, 81.4118) construction
  line L2250 (215.8233, 81.4118) -> (215.7553, 81.2616) construction
  line L2251 (215.7553, 81.2616) -> (215.6863, 81.1115) construction
  line L2252 (215.6863, 81.1115) -> (215.6166, 80.9616) construction
  line L2253 (215.6166, 80.9616) -> (215.5459, 80.8119) construction
  line L2254 (215.5459, 80.8119) -> (215.4745, 80.6624) construction
  line L2255 (215.4745, 80.6624) -> (215.4021, 80.513) construction
  line L2256 (215.4021, 80.513) -> (215.329, 80.3638) construction
  line L2257 (215.329, 80.3638) -> (215.255, 80.2148) construction
  line L2258 (215.255, 80.2148) -> (215.1802, 80.066) construction
  line L2259 (215.1802, 80.066) -> (215.1046, 79.9174) construction
  line L2260 (215.1046, 79.9174) -> (215.0282, 79.7689) construction
  line L2261 (215.0282, 79.7689) -> (214.951, 79.6207) construction
  line L2262 (214.951, 79.6207) -> (214.873, 79.4726) construction
  line L2263 (214.873, 79.4726) -> (214.7942, 79.3248) construction
  line L2264 (214.7942, 79.3248) -> (214.7146, 79.1771) construction
  line L2265 (214.7146, 79.1771) -> (214.6343, 79.0297) construction
  line L2266 (214.6343, 79.0297) -> (214.5531, 78.8824) construction
  line L2267 (214.5531, 78.8824) -> (214.4876, 78.7648) construction
  line L2268 (214.4876, 78.7648) -> (214.4381, 78.6766) construction
  line L2269 (214.4381, 78.6766) -> (214.4049, 78.6179) construction
  line L2270 (214.4049, 78.6179) -> (214.3883, 78.5885) construction
  line L2271 (206.5892, 90.8558) -> (206.4369, 89.2315)
  line L2272 (235.6801, 95.4634) -> (236.3268, 93.9655)
  line L2273 (206.5892, 90.8558) -> (206.4369, 89.2315)
  line L2274 (235.6801, 95.4634) -> (236.3268, 93.9655)
  arc A79 (236.6621, 98.0646) -> (235.6801, 95.4634) centre (237.5162, 96.2562) ccw
  arc A80 (236.6621, 98.0646) -> (235.6801, 95.4634) centre (237.5162, 96.2562) ccw
  spline S30 degree 5 poles (243.2435, 97.4897) (243.2592, 97.4632) (243.2914, 97.4105) (243.3417, 97.3328) (243.4127, 97.2319) (243.5068, 97.1094) (243.6047, 96.9894) (243.7049, 96.8711) (243.8064, 96.7536) (243.9087, 96.6366) (244.012, 96.5203) (244.1164, 96.4049) (244.2223, 96.2906) (244.3301, 96.1776) (244.4397, 96.066) (244.551, 95.9556) (244.6636, 95.8463) (244.7775, 95.7378) (244.8923, 95.6302) (245.008, 95.5233) (245.1247, 95.4172) (245.2425, 95.3119) (245.3612, 95.2074) (245.4811, 95.1039) (245.602, 95.0012) (245.7239, 94.8993) (245.8468, 94.7983) (245.9706, 94.698) (246.0953, 94.5985) (246.2208, 94.4997) (246.3471, 94.4016) (246.4743, 94.3043) (246.6023, 94.2077) (246.7311, 94.1119) (246.8608, 94.0168) (246.9912, 93.9224) (247.1225, 93.8288) (247.2544, 93.7358) (247.3872, 93.6436) (247.5206, 93.552) (247.6548, 93.4612) (247.7897, 93.371) (247.9253, 93.2815) (248.0615, 93.1927) (248.1985, 93.1045) (248.3362, 93.0171) (248.4745, 92.9303) (248.6135, 92.8442) (248.7531, 92.7587) (248.8934, 92.6739) (249.0343, 92.5898) (249.1758, 92.5063) (249.318, 92.4235) (249.4608, 92.3413) (249.6041, 92.2597) (249.7481, 92.1788) (249.8927, 92.0986) (250.0378, 92.019) (250.1835, 91.94) (250.3298, 91.8617) (250.4767, 91.784) (250.6241, 91.7069) (250.7721, 91.6305) (250.9206, 91.5547) (251.0697, 91.4795) (251.2193, 91.405) (251.3694, 91.331) (251.5201, 91.2577) (251.6713, 91.1851) (251.8229, 91.113) (251.9751, 91.0416) (252.0973, 90.9849) (252.1892, 90.9427) (252.2505, 90.9147) (252.2812, 90.9007) knots 0 0 0 0 0 0 0.01428571 0.02857143 0.04285714 0.05714286 0.07142857 0.08571429 0.1 0.11428571 0.12857143 0.14285714 0.15714286 0.17142857 0.18571429 0.2 0.21428571 0.22857143 0.24285714 0.25714286 0.27142857 0.28571429 0.3 0.31428571 0.32857143 0.34285714 0.35714286 0.37142857 0.38571429 0.4 0.41428571 0.42857143 0.44285714 0.45714286 0.47142857 0.48571429 0.5 0.51428571 0.52857143 0.54285714 0.55714286 0.57142857 0.58571429 0.6 0.61428571 0.62857143 0.64285714 0.65714286 0.67142857 0.68571429 0.7 0.71428571 0.72857143 0.74285714 0.75714286 0.77142857 0.78571429 0.8 0.81428571 0.82857143 0.84285714 0.85714286 0.87142857 0.88571429 0.9 0.91428571 0.92857143 0.94285714 0.95714286 0.97142857 0.98571429 1 1 1 1 1 1
  line L2275 (243.2435, 97.4897) -> (243.2592, 97.4632) construction
  line L2276 (243.2592, 97.4632) -> (243.2914, 97.4105) construction
  line L2277 (243.2914, 97.4105) -> (243.3417, 97.3328) construction
  line L2278 (243.3417, 97.3328) -> (243.4127, 97.2319) construction
  line L2279 (243.4127, 97.2319) -> (243.5068, 97.1094) construction
  line L2280 (243.5068, 97.1094) -> (243.6047, 96.9894) construction
  line L2281 (243.6047, 96.9894) -> (243.7049, 96.8711) construction
  line L2282 (243.7049, 96.8711) -> (243.8064, 96.7536) construction
  line L2283 (243.8064, 96.7536) -> (243.9087, 96.6366) construction
  line L2284 (243.9087, 96.6366) -> (244.012, 96.5203) construction
  line L2285 (244.012, 96.5203) -> (244.1164, 96.4049) construction
  line L2286 (244.1164, 96.4049) -> (244.2223, 96.2906) construction
  line L2287 (244.2223, 96.2906) -> (244.3301, 96.1776) construction
  line L2288 (244.3301, 96.1776) -> (244.4397, 96.066) construction
  line L2289 (244.4397, 96.066) -> (244.551, 95.9556) construction
  line L2290 (244.551, 95.9556) -> (244.6636, 95.8463) construction
  line L2291 (244.6636, 95.8463) -> (244.7775, 95.7378) construction
  line L2292 (244.7775, 95.7378) -> (244.8923, 95.6302) construction
  line L2293 (244.8923, 95.6302) -> (245.008, 95.5233) construction
  line L2294 (245.008, 95.5233) -> (245.1247, 95.4172) construction
  line L2295 (245.1247, 95.4172) -> (245.2425, 95.3119) construction
  line L2296 (245.2425, 95.3119) -> (245.3612, 95.2074) construction
  line L2297 (245.3612, 95.2074) -> (245.4811, 95.1039) construction
  line L2298 (245.4811, 95.1039) -> (245.602, 95.0012) construction
  line L2299 (245.602, 95.0012) -> (245.7239, 94.8993) construction
  line L2300 (245.7239, 94.8993) -> (245.8468, 94.7983) construction
  line L2301 (245.8468, 94.7983) -> (245.9706, 94.698) construction
  line L2302 (245.9706, 94.698) -> (246.0953, 94.5985) construction
  line L2303 (246.0953, 94.5985) -> (246.2208, 94.4997) construction
  line L2304 (246.2208, 94.4997) -> (246.3471, 94.4016) construction
  line L2305 (246.3471, 94.4016) -> (246.4743, 94.3043) construction
  line L2306 (246.4743, 94.3043) -> (246.6023, 94.2077) construction
  line L2307 (246.6023, 94.2077) -> (246.7311, 94.1119) construction
  line L2308 (246.7311, 94.1119) -> (246.8608, 94.0168) construction
  line L2309 (246.8608, 94.0168) -> (246.9912, 93.9224) construction
  line L2310 (246.9912, 93.9224) -> (247.1225, 93.8288) construction
  line L2311 (247.1225, 93.8288) -> (247.2544, 93.7358) construction
  line L2312 (247.2544, 93.7358) -> (247.3872, 93.6436) construction
  line L2313 (247.3872, 93.6436) -> (247.5206, 93.552) construction
  line L2314 (247.5206, 93.552) -> (247.6548, 93.4612) construction
  line L2315 (247.6548, 93.4612) -> (247.7897, 93.371) construction
  line L2316 (247.7897, 93.371) -> (247.9253, 93.2815) construction
  line L2317 (247.9253, 93.2815) -> (248.0615, 93.1927) construction
  line L2318 (248.0615, 93.1927) -> (248.1985, 93.1045) construction
  line L2319 (248.1985, 93.1045) -> (248.3362, 93.0171) construction
  line L2320 (248.3362, 93.0171) -> (248.4745, 92.9303) construction
  line L2321 (248.4745, 92.9303) -> (248.6135, 92.8442) construction
  line L2322 (248.6135, 92.8442) -> (248.7531, 92.7587) construction
  line L2323 (248.7531, 92.7587) -> (248.8934, 92.6739) construction
  line L2324 (248.8934, 92.6739) -> (249.0343, 92.5898) construction
  line L2325 (249.0343, 92.5898) -> (249.1758, 92.5063) construction
  line L2326 (249.1758, 92.5063) -> (249.318, 92.4235) construction
  line L2327 (249.318, 92.4235) -> (249.4608, 92.3413) construction
  line L2328 (249.4608, 92.3413) -> (249.6041, 92.2597) construction
  line L2329 (249.6041, 92.2597) -> (249.7481, 92.1788) construction
  line L2330 (249.7481, 92.1788) -> (249.8927, 92.0986) construction
  line L2331 (249.8927, 92.0986) -> (250.0378, 92.019) construction
  line L2332 (250.0378, 92.019) -> (250.1835, 91.94) construction
  line L2333 (250.1835, 91.94) -> (250.3298, 91.8617) construction
  line L2334 (250.3298, 91.8617) -> (250.4767, 91.784) construction
  line L2335 (250.4767, 91.784) -> (250.6241, 91.7069) construction
  line L2336 (250.6241, 91.7069) -> (250.7721, 91.6305) construction
  line L2337 (250.7721, 91.6305) -> (250.9206, 91.5547) construction
  line L2338 (250.9206, 91.5547) -> (251.0697, 91.4795) construction
  line L2339 (251.0697, 91.4795) -> (251.2193, 91.405) construction
  line L2340 (251.2193, 91.405) -> (251.3694, 91.331) construction
  line L2341 (251.3694, 91.331) -> (251.5201, 91.2577) construction
  line L2342 (251.5201, 91.2577) -> (251.6713, 91.1851) construction
  line L2343 (251.6713, 91.1851) -> (251.8229, 91.113) construction